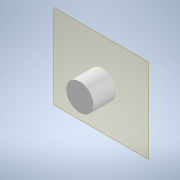
# Autodesk Inventor part: PowerScrew
Saved by Autodesk Inventor 2022 (Build 260153000, 153)
## iProperties
Created: 2022-02-11
Part Number: PowerScrew
Material: Generico
Document SubType Name: Modeling
Designer: matte
Density: 1 g/cm^3
Appearance: Default
Author: matte
Autodesk Inventor part; units mm, degrees
ref_plane "YZ Plane" through (0, 0, 0) normal (1, 0, 0) x (0, 1, 0)
ref_plane "XZ Plane" through (0, 0, 0) normal (0, 1, 0) x (-1, 0, 0)
ref_plane "XY Plane" through (0, 0, 0) normal (0, 0, 1) x (1, 0, 0)
ref_plane "Piano di lavoro1" through (0, 0, 0) normal (0, 0, 1) x (1, 0, 0)
sketch "Schizzo1" plane through (0, 0, 0) normal (0, 0, 1) x (1, 0, 0)
  arc A0 (0.475, -8.4) -> (0.475, 0) centre (0.475, -4.2) ccw projected
  arc A1 (-0.475, 0) -> (-0.475, -8.4) centre (-0.475, -4.2) ccw projected
  line L0 (-0.475, -8.4) -> (0.475, -8.4) projected
  line L1 (0.475, 0) -> (-0.475, 0) projected
  circle A2 centre (0, -4.2) radius 6
  line L2 (0.475, -8.4) -> (-0.475, 0) construction
  line L3 (0.475, 0) -> (-0.475, -8.4) construction
  point P0 (0, 0)
  point P1 (0, -4.2)
  dimension "d0" = 12
  constraints: 4 end point, 1 centre point, 1 coincident, 1 midpoint, 1 point on circle
  measures "d0" diameter of A2
extrude "Estrusione1" add sketch "Schizzo1" along normal blind 587.3 contours L0 A1 L1 A0 | A2
